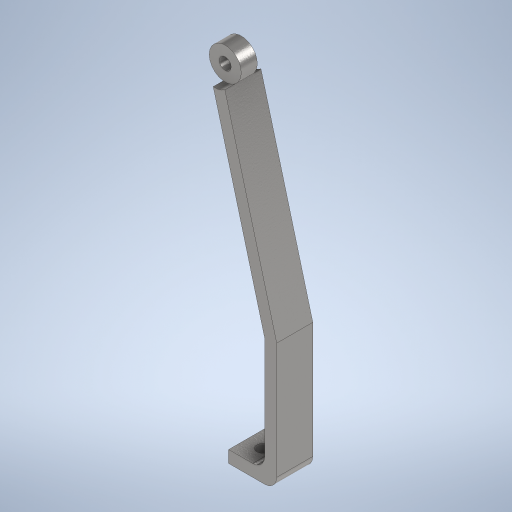
# Autodesk Inventor part: HUDSON-1-73A
Saved by Autodesk Inventor 2024.2 (Build 282272000, 272)
## iProperties
Created: 2024-09-29
Part Number: HUDSON-1-73A
Material: Generic
Document SubType Name: Modeling
Designer: melim
Density: 1 g/cm^3
Appearance: Galvanized
Author: melim
Autodesk Inventor part; units mm, degrees
ref_plane "YZ Plane" through (0, 0, 0) normal (1, 0, 0) x (0, 1, 0)
ref_plane "XZ Plane" through (0, 0, 0) normal (0, 1, 0) x (-1, 0, 0)
ref_plane "XY Plane" through (0, 0, 0) normal (0, 0, 1) x (1, 0, 0)
sketch "Sketch1" plane through (0, 0, 0) normal (0, 0, 1) x (1, 0, 0)
  line L0 (0, 0) -> (0, 31.995)
  line L1 (0, 0) -> (-12, 0)
  line L2 (-12, 0) -> (-12, 3)
  line L3 (-12, 3) -> (-3, 3)
  line L4 (-3, 3) -> (-3, 31.6)
  line L5 (-3, 31.6) -> (-15.941, 79.8963)
  line L6 (-12.944, 80.3028) -> (0, 31.995)
  circle A0 centre (-15.3527, 83.4963) radius 4
  circle A1 centre (-15.3527, 83.4963) radius 1.5
  point P0 (-15.8418, 79.5263)
  dimension "d31" = 8
  dimension "d1" = 3
  dimension "d2" = 3
  dimension "d3" = 9
  dimension "d4" = 28.6
  dimension "d27" = 165
  dimension "d28" = 3
  dimension "d29" = 50
  dimension "d32" = 1.5
  dimension "d34" = 3.6
  dimension "d35" = 3
  constraints: 14 end point, 3 vertical, 2 horizontal, 1 centre point, 1 coincident, 1 parallel, 3 other
  measures "d1" distance of L1.end L2.end
  measures "d2" distance from line of L0 L3.end
  measures "d3" distance of L2.end L3.end
  measures "d4" distance of L3.end L4.end
  measures "d27" angle of L4 L5
  measures "d28" distance between parallel lines of L6 L5
  measures "d29" distance of L4.end L5.end
  measures "d32" distance from line of point (-15.353, 83.496) L5
  measures "d34" vertical distance of L5.end point (-15.353, 83.496)
  measures "d35" diameter of A1
extrude "Extrusion4" add sketch "Sketch1" against normal blind 9 contours L1 L2 L3 L4 L5 A0 L6 L0
extrude "Extrusion5" add sketch "Sketch1" against normal blind 6.5 contours A0
extrude "Extrusion6" cut sketch "Sketch1" against normal blind 2.5 contours A0
sketch "Sketch3" plane through (-12, 3, 0) normal (0, 1, 0) x (1, 0, 0)
  line L0 (0, 0) -> (12, 0) projected
  line L1 (0, 0) -> (0, 9) projected
  line L2 (12, 9) -> (0, 9) projected
  line L3 (12, 0) -> (12, 9) projected
  point P0 (4, 4.5)
  point P1 (0, 4.5)
  dimension "d42" = 4
  dimension "d43" = 4.5
  constraints: 1 midpoint
  measures "d42" distance of point (0, 4.5) point (4, 4.5)
  measures "d43" distance from line of L2 point (4, 4.5)
hole "Hole2" at (-8, 3, -4.5) direction (0, -1, 0) diameter 3 end through all
fillet "Fillet2" radius 3 2 edges at (-3, 3, -4.5) (0, 0, -4.5)
body "Solid2"
